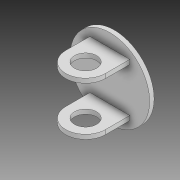
# Autodesk Inventor part: Platform
Saved by Autodesk Inventor 2020 (Build 240168000, 168)
## iProperties
Created: 2021-03-19
Part Number: Platform
Material: Generic
Document SubType Name: Modeling
Designer: DDeGo
Density: 1 g/cm^3
Appearance: Default
Author: DDeGo
Autodesk Inventor part; units mm, degrees
ref_plane "YZ Plane" through (0, 0, 0) normal (1, 0, 0) x (0, 1, 0)
ref_plane "XY Plane" through (0, 0, 0) normal (0, 0, 1) x (1, 0, 0)
sketch "Sketch1" plane through (0, 0, 0) normal (0, 0, 1) x (1, 0, 0)
  circle A0 centre (0, 0) radius 90
  dimension "d0" = 180
  constraints: 1 centre point, 1 coincident
  measures "d0" diameter of A0
extrude "Extrusion1" add sketch "Sketch1" along normal blind 10
ref_plane "Work Plane1" through (0, 50, 0) normal (0, 1, 0) x (-1, 0, 0)
sketch "Sketch2" plane through (0, 50, 0) normal (0, 1, 0) x (-1, 0, 0)
  line L0 (90, 10) -> (-90, 10) projected
  line L1 (0, 10) -> (0, 110) construction
  arc A0 (45, 65) -> (0, 110) centre (0, 65) ccw
  line L2 (45, 65) -> (45, 10)
  line L3 (45, 10) -> (0, 10)
  arc A1 (0, 110) -> (-45, 65) centre (0, 65) ccw
  line L4 (-45, 65) -> (-45, 10)
  line L5 (-45, 10) -> (0, 10)
  circle A2 centre (0, 65) radius 25
  point P0 (0, 0)
  dimension "d4" = 45
  dimension "d5" = 100
  dimension "d6" = 50
  constraints: 10 end point, 4 point on circle, 3 centre point, 2 point on line, 2 symmetric about line, 1 coincident, 1 collinear, 1 midpoint, 1 perpendicular, 1 tangent, 1 vertical, 1 other
  measures "d4" radius of A0
  measures "d5" distance of L1.start L1.end
  measures "d6" diameter of A2
extrude "Extrusion2" add sketch "Sketch2" along normal blind 10
mirror "Mirror1" about plane through (0, 0, 0) normal (0, 1, 0) of "Extrusion2"
body "Solid1"
